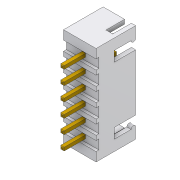
# Autodesk Inventor part: XH-6A
Saved by Autodesk Inventor 2018 (Build 220112000, 112)
## iProperties
Created: 2018-06-15
Part Number: XH-6A
Material: Generic
Document SubType Name: Modeling
Designer: aespen-cad
Density: 1 g/cm^3
Appearance: Default
Author: aespen-cad
Autodesk Inventor part; units mm, degrees
ref_plane "YZ Plane" through (0, 0, 0) normal (1, 0, 0) x (0, 1, 0)
ref_plane "XZ Plane" through (0, 0, 0) normal (0, 1, 0) x (-1, 0, 0)
ref_plane "XY Plane" through (0, 0, 0) normal (0, 0, 1) x (1, 0, 0)
sketch "Sketch1" plane through (0, 0, 0) normal (0, 0, 1) x (1, 0, 0)
  line L0 (0, 7) -> (5.75, 7)
  line L1 (5.75, 7) -> (5.75, 0)
  line L2 (5.75, 0) -> (0, 0)
  line L3 (0, 0) -> (0, 7)
  line L4 (3.8, 7) -> (5, 7)
  line L5 (5, 7) -> (5, 3.7)
  line L6 (5, 3.7) -> (3.8, 3.7)
  line L7 (3.8, 3.7) -> (3.8, 7)
  dimension "d0" = 5.75
  dimension "d1" = 7
  dimension "d2" = 1.2
  dimension "d3" = 3.8
  dimension "d4" = 3.3
  dimension "d5" = 0.75
  constraints: 16 end point, 4 parallel, 2 horizontal, 2 perpendicular, 1 coincident, 1 point on line
  measures "d0" distance of L1.end L2.end
  measures "d1" distance of L0.end L1.end
  measures "d2" distance of L5.end L6.end
  measures "d3" distance between parallel lines of L3 L7
  measures "d4" distance between parallel lines of L0 L6
  measures "d5" distance between parallel lines of L1 L5
extrude "Extrusion2" add sketch "Sketch1" along normal blind 17.4 contours L0 L7 L6 L5 L1 L2 L3
sketch "Sketch2" plane through (0, 7, 0) normal (0, 1, 0) x (1, 0, 0)
  line L0 (5, 0) -> (5, -17.4) projected
  line L1 (0.6, -16.65) -> (5, -16.65)
  line L2 (5, -16.65) -> (5, -0.75)
  line L3 (5, -0.75) -> (0.6, -0.75)
  line L4 (0.6, -0.75) -> (0.6, -16.65)
  line L5 (3.8, -17.4) -> (0, -17.4) projected
  line L6 (3.8, 0) -> (0, 0) projected
  line L7 (0, 0) -> (0, -17.4) projected
  dimension "d10" = 0.75
  dimension "d11" = 0.75
  dimension "d12" = 0.6
  constraints: 8 end point, 2 parallel, 1 horizontal, 1 perpendicular, 1 point on line
  measures "d10" distance between parallel lines of L5 L1
  measures "d11" distance between parallel lines of L3 L6
  measures "d12" distance between parallel lines of L7 L4
extrude "Extrusion3" cut sketch "Sketch2" against normal blind 5.3
sketch "Sketch3" plane through (5.75, 0, 0) normal (1, 0, 0) x (0, 0, -1)
  line L0 (-15.5, 7) -> (-13.7, 7)
  line L1 (-13.7, 7) -> (-13.7, 3.2)
  line L2 (-13.7, 3.2) -> (-15.5, 3.2)
  line L3 (-15.5, 3.2) -> (-15.5, 7)
  line L4 (-17.4, 0) -> (-17.4, 7) projected
  line L5 (0, 7) -> (-17.4, 7) projected
  arc A0 (-15.5, 6.2) -> (-15.5, 7) centre (-15.5, 6.6) ccw
  line L6 (-1.9, 7) -> (-3.7, 7)
  line L7 (-3.7, 7) -> (-3.7, 3.2)
  line L8 (-3.7, 3.2) -> (-1.9, 3.2)
  line L9 (-1.9, 3.2) -> (-1.9, 7)
  line L10 (0, 0) -> (0, 7) projected
  arc A1 (-1.9, 7) -> (-1.9, 6.2) centre (-1.9, 6.6) ccw
  dimension "d15" = 1.8
  dimension "d16" = 1.9
  dimension "d17" = 3.8
  dimension "d18" = 0.8
  dimension "d20" = 1.8
  dimension "d21" = 3.8
  dimension "d22" = 1.9
  dimension "d23" = 0.8
  constraints: 16 end point, 5 point on line, 4 parallel, 4 point on circle, 2 centre point, 2 horizontal, 2 perpendicular, 1 collinear
  measures "d15" distance of L1.end L2.end
  measures "d16" distance between parallel lines of L4 L3
  measures "d17" distance between parallel lines of L0 L2
  measures "d18" distance of L0.start A0.start
  measures "d20" distance of L8.end L7.end
  measures "d21" distance of L7.end L6.end
  measures "d22" distance between parallel lines of L10 L9
  measures "d23" distance of A1.end L6.start
extrude "Extrusion4" cut sketch "Sketch3" against normal blind 1 contours L5 A1 L9 L8 L7 | L0 L1 L2 L3 A0
sketch "Sketch4" plane through (0, 0, 0) normal (0, -1, 0) x (1, 0, 0)
  line L0 (5.75, 0) -> (5.75, 17.4) projected
  line L1 (0, 14.1) -> (5.75, 14.1)
  line L2 (5.75, 14.1) -> (5.75, 15.8)
  line L3 (5.75, 15.8) -> (0, 15.8)
  line L4 (0, 15.8) -> (0, 14.1)
  line L5 (0, 0) -> (0, 17.4) projected
  line L6 (0, 0) -> (5.75, 0) projected
  line L7 (0, 17.4) -> (5.75, 17.4) projected
  dimension "d27" = 1.7
  dimension "d36" = 17.4
  dimension "d43" = 1.6
  constraints: 8 end point, 2 parallel, 1 collinear, 1 horizontal, 1 perpendicular, 1 point on line
  measures "d27" distance between parallel lines of L1 L3
  measures "d36" distance between parallel lines of L6 L7
  measures "d43" distance between parallel lines of L7 L3
extrude "Extrusion5" cut sketch "Sketch4" against normal blind 0.5 contours L1 L4 L3 L0
pattern_linear "Rectangular Pattern2" count 6 spacing 2.5 along (0, 0, -1) of "Extrusion5"
sketch "Sketch5" plane through (0, 0, 17.4) normal (0, -1, 0) x (1, 0, 0)
  line L0 (2.8, -2.15) -> (3.4, -2.15)
  line L1 (3.4, -2.15) -> (3.4, -2.75)
  line L2 (3.4, -2.75) -> (2.8, -2.75)
  line L3 (2.8, -2.75) -> (2.8, -2.15)
  line L4 (0, 0) -> (5.75, 0) projected
  line L5 (5.75, -1.6) -> (5.75, -3.3) projected
  point P0 (0, -17.4)
  dimension "d47" = 0.6
  dimension "d48" = 0.6
  dimension "d49" = 2.15
  dimension "d50" = 2.35
  constraints: 8 end point, 2 parallel, 1 horizontal, 1 perpendicular
  measures "d47" distance of L1.end L2.end
  measures "d48" distance of L0.end L1.end
  measures "d49" distance between parallel lines of L4 L0
  measures "d50" distance between parallel lines of L5 L1
extrude "Extrusion6" add sketch "Sketch5" along normal blind 3.4 and the other way blind 6.1
chamfer "Chamfer1" distance 0.12 angle 45 8 edges at (3.1, -3.4, 15.25) (3.4, -3.4, 14.95) (3.1, -3.4, 14.65) (2.8, -3.4, 14.95) (3.4, 6.1, 14.95) (3.1, 6.1, 15.25) (2.8, 6.1, 14.95) (3.1, 6.1, 14.65)
pattern_linear "Rectangular Pattern3" count 6 spacing 2.5 along (0, 0, -1) of "Extrusion6", "Chamfer1"
equation "\"d11\" = d10"
equation "\"d20\" = d15"
equation "\"d22\" = d16"
equation "\"d23\" = d18"
equation "\"d49\" = 0.5 * d27 + d43 - 0.5 * d48"
body "Solid2"
